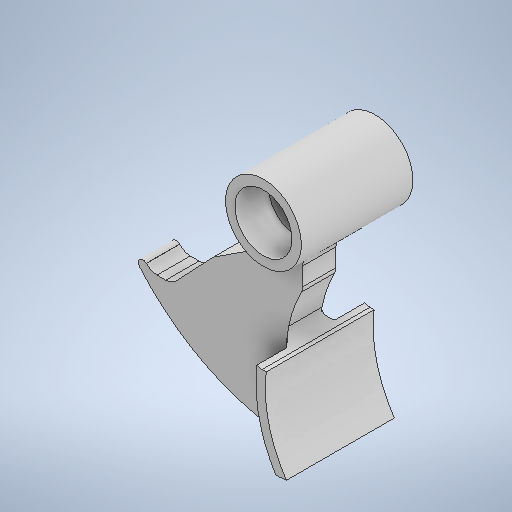
# Autodesk Inventor part: SwingKicker
Saved by Autodesk Inventor 2025.1 (Build 291241000, 241)
## iProperties
Created: 2025-06-11
Part Number: SwingKicker
Material: Generic
Document SubType Name: Modeling
Designer: User
Density: 1 g/cm^3
Appearance: Default
Author: User
## iProperties of the stored document SwingKicker_3DPrint.ipt
Created: 2025-06-15
Part Number: SwingKicker_3DPrint
Material: Generic
Document SubType Name: Modeling
Designer: User
Density: 1 g/cm^3
Appearance: Default
Author: User
Autodesk Inventor part; units mm, degrees
ref_plane "YZ Plane" through (0, 0, 0) normal (1, 0, 0) x (0, 1, 0)
ref_plane "XZ Plane" through (0, 0, 0) normal (0, 1, 0) x (-1, 0, 0)
ref_plane "XY Plane" through (0, 0, 0) normal (0, 0, 1) x (1, 0, 0)
sketch "Sketch1" plane through (0, 0, 0) normal (0, 0, 1) x (1, 0, 0)
  arc A0 (63.773033, 3.219601) -> (63.773033, 3.219601) centre (63.773033, -31.780399) ccw
  line L0 (-5.892521, 0.381945) -> (-8.237485, 0.381945)
  line L1 (-11.093337, 12.599345) -> (-11.093337, 1.686167)
  line L2 (-3.036669, 12.599345) -> (-3.036669, 1.686167)
  line L3 (-7.065003, 0.381945) -> (-7.065003, -1.118055)
  line L4 (-7.065003, -1.118055) -> (-7.065003, -31.118055)
  line L5 (-3.036669, -1.118055) -> (-3.036669, -31.118055)
  line L6 (-11.093337, -1.118055) -> (-11.093337, -31.118055)
  arc A1 (31.00808, -27.848749) -> (36.440717, -50.272141) centre (63.773033, -31.780399) ccw
  circle A2 centre (30.773033, 6.897275) radius 2.6
  circle A3 centre (30.773033, 6.897275) radius 7.65
  arc A4 (37.758913, -0.466147) -> (23.770667, -0.450472) centre (30.773033, 6.897275) ccw
  line L7 (15.492997, 84.008) -> (15.492997, 2.5)
  line L8 (12.492997, 2.5) -> (15.492997, 2.5)
  arc A5 (-11.093337, 1.686167) -> (-8.237485, 0.381945) centre (-8.237485, 4.160781) ccw
  arc A6 (-5.892521, 0.381945) -> (-3.036669, 1.686167) centre (-5.892521, 4.160781) ccw
  line L9 (-5.892521, 0.381945) -> (-8.237485, 0.381945)
  arc A7 (-11.078323, -28.709901) -> (-8.237485, -29.996902) centre (-8.237485, -26.218066) ccw
  arc A8 (-5.892521, -29.996902) -> (-3.036669, -28.69268) centre (-5.892521, -26.218066) ccw
  line L10 (-8.237485, -29.996902) -> (-5.892521, -29.996902)
  arc A9 (-11.078323, -28.709901) -> (-12.983288, -30.330648) centre (-12.018579, -29.534645) ccw
  line L11 (6.841514, -18.294377) -> (23.675208, -7.291301)
  line L12 (23.675208, -7.291301) -> (23.770668, -0.450408)
  line L13 (6.854164, -18.281045) -> (-3.274741, -28.943287)
  line L14 (-3.274741, -28.943287) -> (6.854164, -18.281045)
  line L15 (6.841514, -18.294377) -> (6.854164, -18.281045)
  arc A10 (30.773033, -13.968886) -> (26.508251, -27.586824) centre (63.773033, -31.780399) ccw
  arc A11 (26.508251, -27.586824) -> (31.00808, -27.848749) centre (30.773033, 6.897275) ccw
  arc A12 (-12.983288, -30.330648) -> (31.308694, -50.5505) centre (30.773033, 6.897275) ccw
  arc A13 (-11.103486, -28.682067) -> (-11.093337, -28.69401) centre (30.773033, 6.897275) ccw
  arc A14 (31.308694, -50.5505) -> (36.440717, -50.272141) centre (31.347264, -3.813758) ccw
  line L16 (30.773033, -7.093843) -> (37.758913, -0.466147)
  line L17 (30.773033, -13.968886) -> (30.773033, -7.093843)
  point P0 (0, 0)
  point P1 (-3.036669, -28.69268)
  point P2 (-11.093337, -28.693093)
  dimension "d0" = 1.5
  dimension "d1" = 30
  dimension "d3" = 5.2
  dimension "d4" = 15.3
  dimension "d5" = 2.5
  constraints: 26 point on circle, 24 end point, 14 centre point, 5 vertical, 3 coincident, 3 tangent, 2 point on line, 1 midpoint, 1 vertical alignment, 13 other
  measures "d0" distance of L3.start L3.end
  measures "d1" distance of L3.end L4.end
  measures "d3" diameter of A2
  measures "d4" diameter of A3
  measures "d5" radial gap between concentric circles of A3 A4
extrude "Extrusion1" add sketch "Sketch1" along normal blind 8 contours A11 A1 A14 A0 | A0 A14 A12 A9 A7 L10 A8 L13 L11 L12 A4 L16 L17 A10 A11 | A3 picked at (31.534313, -40.786804)
fillet "Fillet1" radius 3 4 edges at (23.6752, -7.2913, 4) (30.773, -7.0938, 4) (30.773, -13.9689, 4) (26.5083, -27.5868, 4)
sketch "Sketch3" plane through (0, 0, 8) normal (0, 0, 1) x (1, 0, 0)
  arc A0 (30.439699, -14.600792) -> (30.773033, -13.226424) centre (27.773033, -13.226424) ccw
  line L0 (30.773033, -13.226424) -> (30.773033, -8.382966)
  arc A1 (31.708241, -6.206586) -> (30.773033, -8.382966) centre (33.773033, -8.382966) ccw
  line L1 (31.708241, -6.206586) -> (37.758913, -0.466147)
  arc A2 (37.758913, -0.466147) -> (23.770667, -0.450472) centre (30.773033, 6.897275) ccw
  line L2 (23.770667, -0.450472) -> (23.697479, -5.695303)
  arc A3 (22.339146, -8.164597) -> (23.697479, -5.695303) centre (20.697771, -5.653444) ccw
  line L3 (22.339146, -8.164597) -> (6.841514, -18.294377)
  line L4 (6.841514, -18.294377) -> (6.854164, -18.281045)
  line L5 (6.854164, -18.281045) -> (-3.036669, -28.69268)
  arc A4 (-5.892521, -29.996902) -> (-3.036669, -28.69268) centre (-5.892521, -26.218066) ccw
  line L6 (-5.892521, -29.996902) -> (-8.237485, -29.996902)
  arc A5 (-11.078323, -28.709901) -> (-8.237485, -29.996902) centre (-8.237485, -26.218066) ccw
  arc A6 (-11.078323, -28.709901) -> (-11.093337, -28.693093) centre (-12.018579, -29.534645) ccw
  line L7 (-11.093337, -28.693093) -> (-11.093337, -28.69401)
  arc A7 (-11.103486, -28.682067) -> (-11.093337, -28.69401) centre (30.773033, 6.897275) ccw
  arc A8 (-11.103486, -28.682067) -> (-12.983288, -30.330648) centre (-12.018579, -29.534645) ccw
  arc A9 (-12.983288, -30.330648) -> (31.308694, -50.5505) centre (30.773033, 6.897275) ccw
  arc A10 (31.308694, -50.5505) -> (36.440717, -50.272141) centre (31.347264, -3.813758) ccw
  arc A11 (31.00808, -27.848749) -> (36.440717, -50.272141) centre (63.773033, -31.780399) ccw
  arc A12 (29.90334, -27.838659) -> (31.00808, -27.848749) centre (30.773033, 6.897275) ccw
  arc A13 (27.039767, -24.236051) -> (29.90334, -27.838659) centre (29.978428, -24.839599) ccw
  arc A14 (30.439699, -14.600792) -> (27.039767, -24.236051) centre (63.773033, -31.780399) ccw
  circle A15 centre (30.773033, 6.897275) radius 2.6
  point P0 (0, 0)
extrude "Extrusion2" add sketch "Sketch3" along normal blind 0.904
sketch "Sketch4" plane through (0, 0, 8.904) normal (0, 0, 1) x (1, 0, 0)
  arc A0 (31.00808, -27.848749) -> (36.440717, -50.272141) centre (63.773033, -31.780399) ccw
  arc A1 (28.525887, -27.550897) -> (34.370087, -51.67303) centre (63.773033, -31.780399) ccw
  arc A2 (31.308694, -50.5505) -> (36.440717, -50.272141) centre (31.347264, -3.813758) ccw
  arc A3 (27.039767, -24.236051) -> (29.90334, -27.838659) centre (29.978428, -24.839599) ccw
  arc A4 (29.90334, -27.838659) -> (31.00808, -27.848749) centre (30.773033, 6.897275) ccw
  arc A5 (28.535699, -27.469909) -> (33.607126, -50.495849) centre (63.773033, -31.780399) ccw
  point P0 (0, 0)
  point P1 (28.525887, -27.550897)
  dimension "d15" = 2.5
  constraints: 8 point on circle, 2 centre point, 1 concentric
  measures "d15" radial gap between concentric circles of A0 A1
extrude "Extrusion3" add sketch "Sketch4" along normal blind 10
sketch "Sketch5" plane through (0, 0, 0) normal (0, 0, -1) x (-1, 0, 0)
  arc A0 (-31.00808, -27.848749) -> (-29.90334, -27.838659) centre (-30.773033, 6.897275) ccw
  arc A1 (-29.90334, -27.838659) -> (-28.535699, -27.469909) centre (-29.978428, -24.839599) ccw
  arc A2 (-33.607126, -50.495849) -> (-28.535699, -27.469909) centre (-63.773033, -31.780399) ccw
  arc A3 (-36.440717, -50.272141) -> (-33.607126, -50.495849) centre (-31.347264, -3.813758) ccw
  arc A4 (-36.440717, -50.272141) -> (-31.00808, -27.848749) centre (-63.773033, -31.780399) ccw
  point P0 (0, 0)
extrude "Extrusion4" add sketch "Sketch5" along normal blind 10
sketch "Sketch6" plane through (0, 0, 8.904) normal (0, 0, 1) x (1, 0, 0)
  circle A0 centre (30.773033, 6.897275) radius 2.6
  arc A1 (37.758913, -0.466147) -> (23.770667, -0.450472) centre (30.773033, 6.897275) ccw
  circle A2 centre (30.773033, 6.897275) radius 10.15
  point P0 (0, 0)
  point P1 (23.770667, -0.450472)
  constraints: 1 centre point, 1 coincident, 1 concentric
extrude "Extrusion5" add sketch "Sketch6" along normal blind 10.5
sketch "Sketch7" plane through (0, 0, 0) normal (0, 0, -1) x (-1, 0, 0)
  circle A0 centre (-30.773033, 6.897275) radius 10.15
  circle A1 centre (-30.773033, 6.897275) radius 2.6
  point P0 (0, 0)
extrude "Extrusion6" add sketch "Sketch7" along normal blind 10.5
sketch "Sketch8" plane through (30.773033, 6.897275, 19.404) normal (0, 0, 1) x (1, 0, 0)
  circle A0 centre (0, 0) radius 10.15 projected
  circle A1 centre (0, 0) radius 7.65
  point P0 (-30.773033, -6.897275)
  dimension "d24" = 15.3
  constraints: 1 centre point, 1 coincident
  measures "d24" diameter of A1
extrude "Extrusion7" cut sketch "Sketch8" against normal blind 9 contours A1
sketch "Sketch9" plane through (30.773033, 6.897275, -10.5) normal (0, 0, -1) x (-1, 0, 0)
  circle A0 centre (0, 0) radius 7.65 projected
  point P0 (30.773033, -6.897275)
extrude "Extrusion8" cut sketch "Sketch9" against normal blind 9
chamfer "Chamfer4" distance 2 angle 45 3 edges at (28.5308, -27.5104, 8.904) (29.1128, -39.456, 8.904) (29.104, -39.4162, 0)
body "Solid1"
